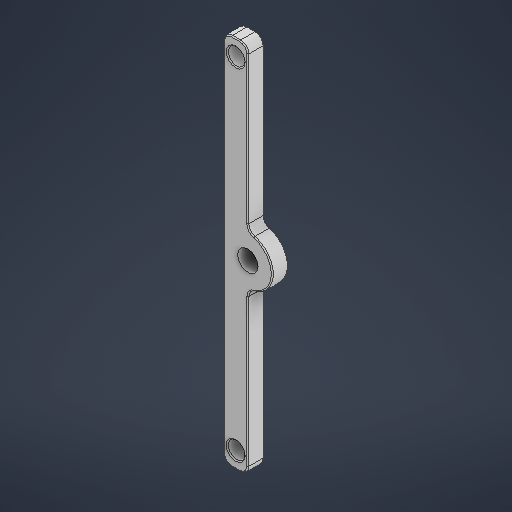
# Autodesk Inventor part: Spacer
Saved by Autodesk Inventor 2026.3 (Build 303398000, 398)
## iProperties
Created: 2026-05-02
Part Number: Spacer
Material: Generic
Document SubType Name: Modeling
Designer: frede
Density: 1 g/cm^3
Appearance: Default
Author: frede
Autodesk Inventor part; units mm, degrees
ref_plane "YZ Plane" through (0, 0, 0) normal (1, 0, 0) x (0, 1, 0)
ref_plane "XZ Plane" through (0, 0, 0) normal (0, 1, 0) x (-1, 0, 0)
ref_plane "XY Plane" through (0, 0, 0) normal (0, 0, 1) x (1, 0, 0)
sketch "Sketch1" plane through (0, 0, 0) normal (0, 0, 1) x (1, 0, 0)
  line L0 (-2, 0) -> (-4, 0)
  line L1 (-6, 2) -> (-6, 90)
  line L2 (-4, 92) -> (-2, 92)
  circle A0 centre (-3, 4) radius 2.075
  circle A1 centre (-3, 88) radius 2.075
  arc A2 (-4, 92) -> (-6, 90) centre (-4, 90) ccw
  arc A3 (0, 90) -> (-2, 92) centre (-2, 90) ccw
  arc A4 (-2, 0) -> (0, 2) centre (-2, 2) ccw
  arc A5 (-6, 2) -> (-4, 0) centre (-4, 2) ccw
  arc A6 (1.5, 40.1905) -> (1.5, 51.8095) centre (0, 46) ccw
  circle A7 centre (0, 46) radius 2.5
  line L3 (0, 90) -> (0, 53.746)
  line L4 (0, 38.254) -> (0, 2)
  arc A8 (0, 53.746) -> (1.5, 51.8095) centre (2, 53.746) ccw
  arc A9 (1.5, 40.1905) -> (0, 38.254) centre (2, 38.254) ccw
  point P0 (0, 0)
  point P1 (-6, 92)
  point P2 (-6, 0)
  point P3 (0, 92)
  point P4 (-3, 92)
  point P5 (0, 40)
  point P6 (0, 52)
  dimension "d0" = 6
  dimension "d1" = 92
  dimension "d2" = 4.15
  dimension "d3" = 4.15
  dimension "d4" = 84
  dimension "d5" = 4
  dimension "d6" = 2
  dimension "d12" = 5
  dimension "d13" = 2
  constraints: 16 point on circle, 14 tangent, 10 centre point, 10 end point, 9 point on line, 4 equal radius, 3 parallel, 1 coincident, 1 horizontal, 1 midpoint, 1 perpendicular
  measures "d0" distance of point (-6, 92) point (0, 92)
  measures "d1" distance of point (-6, 0) point (-6, 92)
  measures "d2" diameter of A0
  measures "d3" diameter of A1
  measures "d4" distance of A0.centre A1.centre
  measures "d5" distance of point (-3, 92) A1.centre
  measures "d6" radius of A2
  measures "d12" diameter of A7
  measures "d13" radius of A8
extrude "Extrusion1" add sketch "Sketch1" along normal blind 4
chamfer "Chamfer1" distance 0.25 angle 45 28 edges at (-5.075, 88, 4) (-5.075, 88, 0) (-3, 92, 0) (-5.4142, 91.4142, 0) (-6, 46, 0) (-5.4142, 0.5858, 0) (-3, 0, 0) (-0.5858, 0.5858, 0) (0, 20.127, 0) (0.4189, 39.4788, 0) (6, 46, 0) (0.4189, 52.5212, 0) (0, 71.873, 0) (-0.5858, 91.4142, 0) (-3, 92, 4) (-5.4142, 91.4142, 4) (-6, 46, 4) (-5.4142, 0.5858, 4) (-3, 0, 4) (-0.5858, 0.5858, 4) (0, 20.127, 4) (0.4189, 39.4788, 4) (6, 46, 4) (0.4189, 52.5212, 4) (0, 71.873, 4) (-0.5858, 91.4142, 4) (-5.075, 4, 4) (-5.075, 4, 0)
equation "\"d3\" = d2"
equation "\"d5\" = -0.5 * d4 + 0.5 * d1"
body "Solid1"
